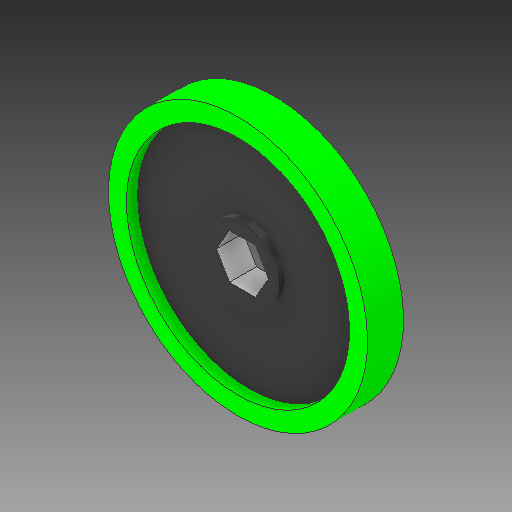
# Autodesk Inventor part: BaneBots_Wheel
Saved by Autodesk Inventor 2018 (Build 220112000, 112)
## iProperties
Created: 2017-04-08
Part Number: BaneBots_Wheel
Material: Generic
Document SubType Name: Modeling
Designer: jklei
Density: 1 g/cm^3
Appearance: Default
Author: jklei
Autodesk Inventor part; units mm, degrees
ref_plane "YZ Plane" through (0, 0, 0) normal (1, 0, 0) x (0, 1, 0)
ref_plane "XZ Plane" through (0, 0, 0) normal (0, 1, 0) x (-1, 0, 0)
ref_plane "XY Plane" through (0, 0, 0) normal (0, 0, 1) x (1, 0, 0)
sketch "Sketch1" plane through (0, 0, 0) normal (1, 0, 0) x (0, 1, 0)
  line L0 (0, -10.16) -> (0, -1.27)
  line L1 (0, -1.27) -> (0, -8.89)
  line L2 (0, -1.27) -> (-10.16, -1.27)
  line L3 (-10.16, -8.89) -> (0, -8.89)
  line L4 (0, -8.89) -> (0, -1.27)
  line L5 (-31.4325, -3.175) -> (-10.16, -3.175)
  line L6 (-10.16, -6.985) -> (-31.4325, -6.985)
  line L7 (-10.16, -1.27) -> (-10.16, -3.175)
  line L8 (-10.16, -6.985) -> (-10.16, -8.89)
  line L9 (-31.4325, -3.175) -> (-31.4325, 0)
  line L10 (-31.4325, 0) -> (-36.5125, 0)
  line L11 (-36.5125, 0) -> (-36.5125, -10.16)
  line L12 (-31.4325, -6.985) -> (-31.4325, -10.16)
  line L13 (-31.4325, -10.16) -> (-36.5125, -10.16)
  point P0 (0, 0)
  dimension "d11" = 10.16
  dimension "d16" = 21.2725
  dimension "d17" = 21.2725
  dimension "d18" = 5.08
  dimension "d19" = 10.16
  constraints: 28 end point, 5 perpendicular, 4 parallel, 2 horizontal, 2 vertical, 1 point on line
  measures "d11" distance of L1.end L3.start
  measures "d16" distance of L5.start L5.end
  measures "d17" distance of L6.start L6.end
  measures "d18" distance of L9.end L10.end
  measures "d19" distance of L10.end L11.end
revolve "Revolution1" add sketch "Sketch1" angle 360 about axis through (0, 0, -10.16) along (0, 0, 1)
sketch "Sketch2" plane through (0, 0, -1.27) normal (0, 0, 1) x (1, 0, 0)
  line L0 (0, 0) -> (0, 6.35)
  line L1 (3.6662, 6.35) -> (7.3323, 0)
  line L2 (7.3323, 0) -> (3.6662, -6.35)
  line L3 (3.6662, -6.35) -> (-3.6662, -6.35)
  line L4 (-3.6662, -6.35) -> (-7.3323, 0)
  line L5 (-7.3323, 0) -> (-3.6662, 6.35)
  line L6 (-3.6662, 6.35) -> (3.6662, 6.35)
  dimension "d12" = 6.35
  constraints: 14 end point, 2 coincident, 1 vertical, 13 other
  measures "d12" distance of L0.start L0.end
extrude "Extrusion1" cut sketch "Sketch2" against normal blind 25.4
body "Solid1"
